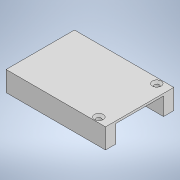
# Autodesk Inventor part: Стойка под электроннику
Saved by Autodesk Inventor 2020 (Build 240168000, 168)
## iProperties
Created: 2021-04-05
Part Number: Стойка под электроннику
Material: Типовые
Document SubType Name: Обычные детали
Designer: Антон
Density: 1 g/cm^3
Appearance: По умолчанию
Sheet Metal Rule: По умолчанию
Author: Антон
Autodesk Inventor part; units mm, degrees
ref_plane "YZ Plane" through (0, 0, 0) normal (1, 0, 0) x (0, 1, 0)
ref_plane "XZ Plane" through (0, 0, 0) normal (0, 1, 0) x (-1, 0, 0)
ref_plane "XY Plane" through (0, 0, 0) normal (0, 0, 1) x (1, 0, 0)
sketch "Эскиз1" plane through (0, 0, 0) normal (0, 1, 0) x (-1, 0, 0)
  line L0 (0, 0) -> (66.9, 0)
  line L1 (66.9, 0) -> (66.9, -46)
  line L2 (66.9, -46) -> (0, -46)
  line L3 (0, -46) -> (0, 0)
  line L4 (61.9, -7) -> (0, -7)
  line L5 (0, -7) -> (0, -39)
  line L6 (0, -39) -> (61.9, -39)
  line L7 (61.9, -39) -> (61.9, -7)
  line L8 (61.9, -7) -> (0, -39) construction
  line L9 (0, -7) -> (61.9, -39) construction
  line L10 (0, -7) -> (2, -7)
  point P0 (0, -7)
  dimension "d0" = 66.9
  dimension "d224" = 7
  dimension "d225" = 5
  dimension "d226" = 32
  dimension "d302" = 7
  constraints: 22 end point, 4 parallel, 3 horizontal, 2 perpendicular, 1 point on line
  measures "d0" distance of L1.end L2.end
  measures "d224" distance between parallel lines of L0 L4
  measures "d225" distance between parallel lines of L1 L7
  measures "d226" distance between parallel lines of L6 L4
  measures "d302" distance between parallel lines of L2 L6
extrude "Выдавливание1" add sketch "Эскиз1" along normal blind 12 contours L0 L1 L2 L3 L6 L7 L4
sketch "Эскиз40" plane through (0, 12, 0) normal (0, 1, 0) x (1, 0, 0)
  line L0 (0, 46) -> (-66.9, 46) projected
  line L1 (0, 0) -> (-66.9, 0)
  line L2 (-66.9, 0) -> (-66.9, 46)
  line L3 (-66.9, 46) -> (0, 46)
  line L4 (0, 46) -> (0, 0)
  constraints: 8 end point, 2 parallel, 1 horizontal, 1 perpendicular
extrude "Выдавливание32" add sketch "Эскиз40" along normal blind 1.5
sketch "Эскиз39" plane through (0, 13.5, 0) normal (0, 1, 0) x (1, 0, 0)
  line L0 (0, 0) -> (0, 7) projected
  line L1 (0, 3.5) -> (-8, 3.5)
  line L2 (0, 42.5) -> (-8, 42.5)
  line L3 (0, 39) -> (0, 46) projected
  dimension "d303" = 8
  constraints: 4 end point, 2 horizontal, 2 midpoint, 1 parallel
  measures "d303" distance of L1.start L1.end
hole "Отверстие6" at (-8, 13.5, -3.5) at (-8, 13.5, -42.5) direction (0, -1, 0) diameter 3.2 end through all countersink diameter 6 countersink angle 90
sketch "Эскиз30" plane through (0, 0, 0) normal (0, -1, 0) x (1, 0, 0)
  line L0 (-66.9, -36.85) -> (-64.9, -36.85)
  line L1 (-64.9, -36.85) -> (-64.9, -9.15)
  line L2 (-64.9, -9.15) -> (-66.9, -9.15)
  line L3 (-66.9, -9.15) -> (-66.9, -36.85)
  line L4 (-66.9, -46) -> (-66.9, 0) projected
  line L5 (-64.9, -36.85) -> (-66, -36.85)
  line L6 (-66, -36.85) -> (-66, -37.85)
  line L7 (-66, -37.85) -> (-64.9, -37.85)
  line L8 (-64.9, -37.85) -> (-64.9, -36.85)
  line L9 (-64.9, -9.15) -> (-66.4, -9.15)
  line L10 (-66.4, -9.15) -> (-66.4, -8.15)
  line L11 (-66.4, -8.15) -> (-64.9, -8.15)
  line L12 (-64.9, -8.15) -> (-64.9, -9.15)
  point P0 (0, 0)
  point P1 (-66.9, -23)
  point P2 (-66.4, -9.15)
  dimension "d216" = 27.7
  dimension "d217" = 2
  dimension "d218" = 1.1
  dimension "d219" = 1
  dimension "d220" = 1.5
  dimension "d221" = 1
  constraints: 24 end point, 6 parallel, 3 horizontal, 3 perpendicular, 2 midpoint
  measures "d216" distance of L0.end L1.end
  measures "d217" distance of L0.start L0.end
  measures "d218" distance of L7.end L6.end
  measures "d219" distance of L7.end L0.end
  measures "d220" distance of L10.end L11.end
  measures "d221" distance of L9.end L10.end
extrude "Выдавливание24" cut sketch "Эскиз30" against normal blind 13.1
